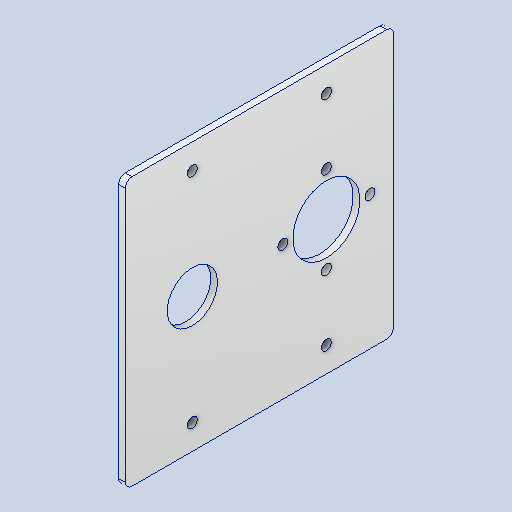
# Autodesk Inventor part: ball_loading_v1_Plate_left_down_M_F
Saved by Autodesk Inventor 2025.1 (Build 291241000, 241)
## iProperties
Created: 2024-11-12
Part Number: ball_loading_v1_Plate_left_down_M_F
Material: アルミニウム 6061
Document SubType Name: Modeling
Designer: haruy
Density: 2.7 g/cm^3
Appearance: アルミニウム - フラット
Author: haruy
Autodesk Inventor part; units mm, degrees
ref_plane "YZ Plane" through (0, 0, 0) normal (1, 0, 0) x (0, 1, 0)
ref_plane "XZ Plane" through (0, 0, 0) normal (0, 1, 0) x (-1, 0, 0)
ref_plane "XY Plane" through (0, 0, 0) normal (0, 0, 1) x (1, 0, 0)
derived "ball_loading_v1_Sketch_Base.ipt"
sketch "スケッチ3" plane through (200, 0, 0) normal (1, 0, 0) x (0, 1, 0)
  line L0 (0, 0) -> (360, 0)
  line L1 (360, 0) -> (360, -15)
  line L2 (360, -15) -> (0, -15)
  line L3 (0, -15) -> (0, 0)
  line L4 (0, 35) -> (-15, 35)
  line L5 (-15, 35) -> (-15, -192.5)
  line L6 (-15, -192.5) -> (0, -192.5)
  line L7 (0, -192.5) -> (0, 35)
  line L8 (0, 35) -> (-15, 35)
  line L9 (-15, 35) -> (-15, 20)
  line L10 (-15, 20) -> (0, 20)
  line L11 (0, 20) -> (0, 35)
  line L12 (50, -15) -> (65, -15)
  line L13 (65, -15) -> (65, -192.5)
  line L14 (65, -192.5) -> (50, -192.5)
  line L15 (50, -192.5) -> (50, -15)
  line L16 (360, -15) -> (345, -15)
  line L17 (345, -15) -> (345, -192.5)
  line L18 (345, -192.5) -> (360, -192.5)
  line L19 (360, -192.5) -> (360, -15)
  circle A0 centre (25, -60) radius 12.5
  circle A1 centre (25, -100) radius 18.75
  line L20 (360, -192.5) -> (0, -192.5)
  line L21 (-15, -40) -> (65, -40)
  line L22 (65, -120) -> (-15, -120)
  circle A2 centre (25, -100) radius 20
  line L23 (42.5, 0) -> (42.5, -15)
  line L24 (65, -15) -> (65, 0)
  line L25 (20, 0) -> (20, -15)
  line L26 (0, 7.5) -> (-15, 7.5)
  line L27 (0, -22.5) -> (-15, -22.5)
  circle A3 centre (325, -60) radius 12.5
  line L28 (360, -35) -> (345, -35)
  line L29 (337.5, 0) -> (337.5, -15)
  line L30 (0, -385) -> (360, -385)
  line L31 (360, -370) -> (0, -370)
  line L32 (0, -370) -> (0, -385)
  circle A4 centre (25, -325) radius 12.5
  line L33 (-15, -345) -> (65, -345)
  line L34 (0, -362.5) -> (-15, -362.5)
  line L35 (50, -370) -> (65, -370)
  line L36 (65, -370) -> (65, -385)
  line L37 (42.5, -385) -> (42.5, -370)
  line L38 (20, -385) -> (20, -370)
  line L39 (65, -265) -> (-15, -265)
  circle A5 centre (25, -285) radius 18.75
  circle A6 centre (25, -285) radius 20
  line L40 (65, -370) -> (65, -192.5)
  line L41 (50, -192.5) -> (50, -370)
  line L42 (0, -192.5) -> (0, -420)
  line L43 (-15, -420) -> (-15, -192.5)
  line L44 (0, -420) -> (-15, -420)
  line L45 (337.5, -385) -> (337.5, -370)
  line L46 (360, -370) -> (345, -370)
  line L47 (360, -385) -> (360, -370)
  line L48 (360, -350) -> (345, -350)
  line L49 (345, -370) -> (345, -192.5)
  line L50 (360, -192.5) -> (360, -370)
  circle A7 centre (325, -325) radius 12.5
  line L51 (0, -420) -> (-15, -420)
  line L52 (-15, -420) -> (-15, -405)
  line L53 (-15, -405) -> (0, -405)
  line L54 (0, -405) -> (0, -420)
  line L55 (0, -392.5) -> (-15, -392.5)
  line L56 (360, -40) -> (312.5, -40)
  line L57 (312.5, -40) -> (312.5, -120)
  line L58 (312.5, -120) -> (360, -120)
  line L59 (360, -120) -> (360, -40)
  line L60 (345, -40) -> (320.9774, -48.1649)
  line L61 (314.1566, -66.2186) -> (345, -120)
  circle A8 centre (25, -60) radius 7.5
  circle A9 centre (25, -100) radius 10
  circle A10 centre (25, -100) radius 13
  circle A11 centre (38, -100) radius 1.5
  circle A12 centre (25, -87) radius 1.5
  circle A13 centre (12, -100) radius 1.5
  circle A14 centre (25, -113) radius 1.5
  circle A15 centre (57.5, -60) radius 1.5
  circle A16 centre (57.5, -100) radius 1.5
  circle A17 centre (-7.5, -100) radius 1.5
  circle A18 centre (-7.5, -60) radius 1.5
  circle A19 centre (57.5, -90) radius 1.5
  circle A20 centre (57.5, -50) radius 1.5
  line L62 (59, -50) -> (59, -60)
  line L63 (56, -50) -> (56, -60)
  line L64 (59, -90) -> (59, -100)
  line L65 (56, -100) -> (56, -90)
  line L66 (25, -40) -> (25, -120)
  circle A21 centre (-7.5, -90) radius 1.5
  circle A22 centre (-7.5, -50) radius 1.5
  line L67 (-9, -50) -> (-9, -60)
  line L68 (-6, -50) -> (-6, -60)
  line L69 (-9, -90) -> (-9, -100)
  line L70 (-6, -100) -> (-6, -90)
  point P0 (352.5, -60)
  point P1 (352.5, -100)
  point P2 (345, -103.75)
  point P3 (-6, -60)
  point P4 (-6, -100)
  dimension "d3" = 26
  dimension "d1" = 15
  dimension "d2" = 20
  dimension "d4" = 3
  dimension "d7" = 360
  dimension "d9" = 20
  dimension "d10" = 20
  dimension "d11" = 20
  dimension "d12" = 20
  dimension "d13" = 7.5
  dimension "d14" = 7.5
  dimension "d15" = 7.5
  dimension "d16" = 7.5
  dimension "d17" = 3
  dimension "d18" = 3
  dimension "d19" = 3
  dimension "d20" = 3
  dimension "d21" = 3
  dimension "d22" = 3
  dimension "d23" = 10
  dimension "d24" = 7.5
  dimension "d25" = 10
  measures "d1" diameter of A8
  measures "d2" diameter of A9
  measures "d4" diameter of A11
  measures "d9" distance from line of point (-7.5, -100) L22
  measures "d10" distance from line of L21 point (-7.5, -60)
  measures "d11" distance from line of point (57.5, -60) L21
  measures "d12" distance from line of L22 point (57.5, -100)
  measures "d13" distance from line of L13 point (57.5, -60)
  measures "d14" distance from line of L13 point (57.5, -100)
  measures "d15" distance from line of point (-7.5, -60) L5
  measures "d16" distance from line of point (-7.5, -100) L5
  measures "d17" diameter of A15
  measures "d18" diameter of A16
  measures "d19" diameter of A17
  measures "d20" diameter of A18
  measures "d21" diameter of A19
  measures "d22" diameter of A20
  measures "d23" distance of A15.centre A20.centre
  measures "d24" distance from line of L13 A20.centre
  measures "d25" distance of A16.centre A19.centre
ref_plane "作業平面1" through (200, 0, 0) normal (1, 0, 0) x (0, 1, 0)
ref_plane "作業平面2" through (0, 0, 200) normal (0, 0, 1) x (1, 0, 0)
extrude "押し出し1" add sketch "スケッチ3" along normal blind 2 contours L21 L66 A0 A2 L22 L7 | L7 L22 L5 L21 | L21 L15 L22 A2 L66 A0 | L13 L22 L15 L21 | L66 A1 A2 | A2 L66 A1 | L66 A8 A0 | A0 L66 A8 | L66 A14 A10 A11 A12 A1 | A1 L66 A12 A10 A13 A14 | A10 A13 A12 L66 A9 A14 | L66 A9 A12 A10 A11 A14 | A15 L63 A20 L62 | A20 | A16 L65 A19 L64 | A19 | A17 L69 A21 L70 | A21 | A18 L67 A22 L68 | A22
fillet "フィレット1" radius 2 4 edges at (201, 65, -40) (201, -15, -40) (201, -15, -120) (201, 65, -120)
sketch "スケッチ2" plane through (0, 0, 200) normal (0, 0, 1) x (1, 0, 0)
  line L0 (0, 0) -> (-15, 0) projected
  line L1 (-15, 0) -> (-15, 248.5284) projected
  line L2 (-15, 248.5284) -> (0, 248.5284) projected
  line L3 (0, 248.5284) -> (0, 0) projected
  line L4 (-320, 0) -> (-305, 0) projected
  line L5 (-305, 0) -> (-305, 238.0267) projected
  line L6 (-305, 238.0267) -> (-320, 238.0267) projected
  line L7 (-320, 238.0267) -> (-320, 0) projected
  line L8 (-320, 0) -> (-324, 0) projected
  line L9 (-324, 0) -> (-324, 76.8713) projected
  line L10 (-324, 76.8713) -> (-320, 76.8713) projected
  line L11 (-320, 76.8713) -> (-320, 0) projected
  line L12 (-15, 0) -> (-19, 0) projected
  line L13 (-19, 0) -> (-19, 51.1976) projected
  line L14 (-19, 51.1976) -> (-15, 51.1976) projected
  line L15 (-15, 51.1976) -> (-15, 0) projected
  line L16 (-335, 13.6956) -> (-4, 13.6956) projected
  line L17 (-4, 13.6956) -> (-4, 23.6956) projected
  line L18 (-4, 23.6956) -> (-335, 23.6956) projected
  line L19 (-335, 23.6956) -> (-335, 13.6956) projected
  line L20 (-216, 31.1956) -> (-114, 31.1956) projected
  line L21 (-114, 31.1956) -> (-114, 6.1956) projected
  line L22 (-114, 6.1956) -> (-216, 6.1956) projected
  line L23 (-216, 6.1956) -> (-216, 31.1956) projected
  line L24 (-150, 31.1956) -> (-146, 31.1956) projected
  line L25 (-146, 31.1956) -> (-146, 6.1956) projected
  line L26 (-146, 6.1956) -> (-150, 6.1956) projected
  line L27 (-150, 6.1956) -> (-150, 31.1956) projected
  line L28 (-198, 31.1956) -> (-194, 31.1956) projected
  line L29 (-194, 31.1956) -> (-194, 6.1956) projected
  line L30 (-194, 6.1956) -> (-198, 6.1956) projected
  line L31 (-198, 6.1956) -> (-198, 31.1956) projected
  line L32 (-126, 31.1956) -> (-122, 31.1956) projected
  line L33 (-122, 31.1956) -> (-122, 6.1956) projected
  line L34 (-122, 6.1956) -> (-126, 6.1956) projected
  line L35 (-126, 6.1956) -> (-126, 31.1956) projected
  circle A0 centre (-165.0738, 76.8713) radius 120 projected
  line L36 (-174, 31.1956) -> (-170, 31.1956) projected
  line L37 (-170, 31.1956) -> (-170, 6.1956) projected
  line L38 (-170, 6.1956) -> (-174, 6.1956) projected
  line L39 (-174, 6.1956) -> (-174, 31.1956) projected
  line L40 (-160, 31.1956) -> (-160, 6.1956) projected
equation "\"d10\" = d9"
equation "\"d11\" = d9"
equation "\"d12\" = d9"
equation "\"d14\" = d13"
equation "\"d15\" = d13"
equation "\"d16\" = d13"
equation "\"d24\" = d13"
